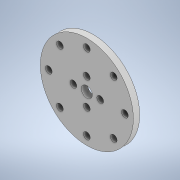
# Autodesk Inventor part: fixation_circle
Saved by Autodesk Inventor 2022 (Build 260153000, 153)
## iProperties
Created: 2022-01-31
Part Number: fixation_circle
Material: Generic
Document SubType Name: Modeling
Designer: Martijn
Density: 1 g/cm^3
Appearance: Default
Author: Martijn
Autodesk Inventor part; units mm, degrees
ref_plane "YZ Plane" through (0, 0, 0) normal (1, 0, 0) x (0, 1, 0)
ref_plane "XZ Plane" through (0, 0, 0) normal (0, 1, 0) x (-1, 0, 0)
ref_plane "XY Plane" through (0, 0, 0) normal (0, 0, 1) x (1, 0, 0)
sketch "Sketch1" plane through (0, 0, 0) normal (0, 0, 1) x (1, 0, 0)
  circle A0 centre (0, 0) radius 22
  circle A1 centre (0, 0) radius 2.6
  dimension "d0" = 44
  dimension "d3" = 5.2
  constraints: 2 centre point, 2 coincident
  measures "d0" diameter of A0
  measures "d3" diameter of A1
extrude "Extrusion1" add sketch "Sketch1" along normal blind 3
sketch "Sketch2" plane through (0, 0, 3) normal (0, 0, 1) x (1, 0, 0)
  circle A0 centre (-6.35, 0) radius 1.6
  point P0 (0, 0)
  dimension "d4" = 3.2
  dimension "d5" = 6.35
  constraints: 1 centre point
  measures "d4" diameter of A0
  measures "d5" distance of point (0, 0) A0.centre
extrude "Extrusion2" cut sketch "Sketch2" against normal blind 3
pattern_circular "Circular Pattern1" count 4 over 360 about axis through (0, 0, 0) along (0, 0, 1) of "Extrusion2"
sketch "Sketch3" plane through (0, 0, 3) normal (0, 0, 1) x (1, 0, 0)
  circle A0 centre (-18, 0) radius 1.6
  circle A1 centre (0, 0) radius 2.6 projected
  line L0 (-18, 0) -> (0, 0)
  line L1 (-30.8, 0) -> (30.8, 0) projected
  dimension "d11" = 3.2
  dimension "d12" = 18
  constraints: 1 centre point, 1 horizontal, 1 horizontal alignment, 2 other
  measures "d11" diameter of A0
  measures "d12" distance of A1.centre A0.centre
extrude "Extrusion3" cut sketch "Sketch3" against normal blind 3 contours L0 L1 A0 | A0 L1 L0
pattern_circular "Circular Pattern2" count 8 over 360 about axis through (0, 0, 0) along (0, 0, 1) of "Extrusion3"
body "Solid1"
